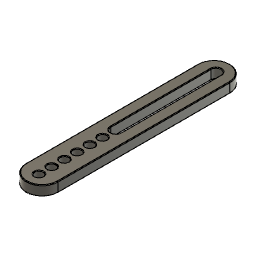
B913F (Autodesk Fusion 360 design; units mm, degrees)
Autodesk Fusion 360 part; units mm, degrees
sketch "Esboço1" plane through (0, 0, 0) normal (0, 1, 0) x (1, 0, 0)
  line L0 (0, 7.9375) -> (0, 93.6625)
  line L1 (15.875, 93.6625) -> (15.875, 7.9375)
  arc A0 (0, 7.9375) -> (15.875, 7.9375) centre (7.9375, 7.9375) ccw
  arc A1 (15.875, 93.6625) -> (0, 93.6625) centre (7.9375, 93.6625) ccw
  line L2 (7.9375, 38.1) -> (7.9375, 38)
  line L3 (7.9375, 6.35) -> (7.9375, 7.9375)
  circle A2 centre (7.9375, 6.35) radius 2.108
  circle A3 centre (7.9375, 12.7) radius 2.108
  circle A4 centre (7.9375, 19.05) radius 2.108
  circle A5 centre (7.9375, 25.4) radius 2.108
  circle A6 centre (7.9375, 31.75) radius 2.108
  circle A7 centre (7.9375, 38.1) radius 2.108
  line L4 (7.9375, 12.7) -> (7.9375, 14.808)
  arc A8 (10.4775, 94.767) -> (5.3975, 94.767) centre (7.9375, 94.767) ccw
  arc A9 (5.3975, 44.704) -> (10.4775, 44.704) centre (7.9375, 44.704) ccw
  line L5 (5.3975, 94.767) -> (5.3975, 44.704)
  line L6 (10.4775, 94.767) -> (10.4775, 44.704)
  dimension "d7" = 6.35
  dimension "d8" = 6.35
  dimension "d9" = 6.35
  dimension "d10" = 6.35
  dimension "d11" = 6.35
  dimension "d12" = 4.216
  dimension "d13" = 4.216
  dimension "d14" = 4.216
  dimension "d15" = 4.216
  dimension "d16" = 4.216
  dimension "d17" = 4.216
  dimension "d19" = 5.08
  dimension "d20" = 50.063
  dimension "d21" = 5.08
  constraint vertical L0
  constraint coincident A0.centre L3.end
  constraint coincident L3.start A2.centre
  constraint coincident A3.centre L4.start
  constraint coincident L2.start A7.centre
  constraint coincident A3 L4.end
  constraint tangent A9 L5
  measures "d7" distance of L3.start A3.centre
  measures "d8" distance of A3.centre A4.centre
  measures "d9" distance of A4.centre A5.centre
  measures "d10" distance of A5.centre A6.centre
  measures "d11" distance of L2.start A6.centre
  measures "d12" diameter of A2
  measures "d13" diameter of A3
  measures "d14" diameter of A4
  measures "d15" diameter of A5
  measures "d16" diameter of A6
  measures "d17" diameter of A7
  measures "d19" diameter of A8
  measures "d20" distance of A8.centre A9.centre
  measures "d21" diameter of A9
extrude "Extrusão1" add sketch "Esboço1" along normal blind 4.699
chamfer "Chanfro1" distance 0.3 angle 45 14 edges at (15.875, 4.699, -50.8) (7.9375, 4.699, -101.6) (0, 4.699, -50.8) (7.9375, 4.699, 0) (10.4775, 4.699, -69.7355) (7.9375, 4.699, -42.164) (5.3975, 4.699, -69.7355) (7.9375, 4.699, -97.307) (5.9722, 4.699, -38.8623) (5.9722, 4.699, -32.5123) (5.9722, 4.699, -26.1623) (5.9722, 4.699, -19.8123) (5.9722, 4.699, -13.4623) (5.9722, 4.699, -7.1123)
